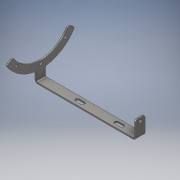
# Autodesk Inventor part: Bellmouth_union
Saved by Autodesk Inventor 2019 (Build 230136000, 136)
## iProperties
Created: 2021-06-28
Part Number: Bellmouth_union
Material: Stainless Steel
Document SubType Name: Sheet Metal
Designer: rtavi
Density: 8 g/cm^3
Sheet Metal Rule: Default_mm
Appearance: Semi-Polished
Mass: 21.766 g
Surface Area: 44.0313 cm^2
Volume: 2.72075 cm^3
Author: rtavi
Autodesk Inventor part; units mm, degrees
ref_plane "YZ Plane" through (0, 0, 0) normal (1, 0, 0) x (0, 1, 0)
ref_plane "XZ Plane" through (0, 0, 0) normal (0, 1, 0) x (-1, 0, 0)
ref_plane "XY Plane" through (0, 0, 0) normal (0, 0, 1) x (1, 0, 0)
sketch "Sketch1" plane through (0, 0, 0) normal (0, 1, 0) x (-1, 0, 0)
  arc A0 (33.3436, 28.8878) -> (33.3436, -28.8878) centre (52.2049, 0) ccw
  arc A1 (29.1632, 35.7118) -> (10.234, 6.6854) centre (52.2049, 0) ccw
  line L0 (33.9823, 31.5624) -> (31.9796, 35.0312)
  line L1 (33.9823, -31.5624) -> (31.9796, -35.0312)
  line L2 (134.5287, 0) -> (-168.388, 0) construction
  line L3 (8.2589, 5) -> (-106.7, 5)
  line L4 (-106.7, 5) -> (-106.7, -5) construction
  line L5 (-106.7, -5) -> (8.2589, -5)
  arc A2 (10, 5) -> (10, -5) centre (52.2049, 0) ccw construction
  arc A3 (10.234, -6.6854) -> (29.1632, -35.7118) centre (52.2049, 0) ccw
  circle A4 centre (14.7049, 0) radius 1.55
  circle A5 centre (25.6884, -26.5165) radius 1.55
  circle A6 centre (52.2049, -37.5) radius 1.55
  circle A7 centre (78.7214, -26.5165) radius 1.55
  circle A8 centre (89.7049, 0) radius 1.55
  circle A9 centre (78.7214, 26.5165) radius 1.55
  circle A10 centre (52.2049, 37.5) radius 1.55
  circle A11 centre (25.6884, 26.5165) radius 1.55
  line L6 (-82.1, -2.1) -> (-87.9, -2.1)
  line L7 (-90, 0) -> (-90, 0)
  line L8 (-87.9, 2.1) -> (-82.1, 2.1)
  line L9 (-80, 0) -> (-80, 0)
  arc A12 (-80, 0) -> (-82.1, 2.1) centre (-82.1, 0) ccw
  arc A13 (-82.1, -2.1) -> (-80, 0) centre (-82.1, 0) ccw
  arc A14 (-90, 0) -> (-87.9, -2.1) centre (-87.9, 0) ccw
  arc A15 (-87.9, 2.1) -> (-90, 0) centre (-87.9, 0) ccw
  arc A16 (-106.7, -3) -> (-104.7, -5) centre (-104.7, -3) ccw construction
  arc A17 (-104.7, 5) -> (-106.7, 3) centre (-104.7, 3) ccw construction
  arc A18 (29.1632, -35.7118) -> (31.9796, -35.0312) centre (30.2475, -34.0312) ccw
  arc A19 (33.9823, -31.5624) -> (33.3436, -28.8878) centre (32.2502, -30.5624) ccw
  arc A20 (33.3436, 28.8878) -> (33.9823, 31.5624) centre (32.2502, 30.5624) ccw
  arc A21 (31.9796, 35.0312) -> (29.1632, 35.7118) centre (30.2475, 34.0312) ccw
  arc A22 (8.2589, 5) -> (10.234, 6.6854) centre (8.2589, 7) ccw
  arc A23 (10.234, -6.6854) -> (8.2589, -5) centre (8.2589, -7) ccw
  line L10 (-47.6, 0) -> (-47.6, 0)
  arc A24 (-47.6, 0) -> (-45.5, -2.1) centre (-45.5, 0) ccw
  arc A25 (-45.5, 2.1) -> (-47.6, 0) centre (-45.5, 0) ccw
  line L11 (-37.6, 0) -> (-37.6, 0)
  arc A26 (-37.6, 0) -> (-39.7, 2.1) centre (-39.7, 0) ccw
  arc A27 (-39.7, -2.1) -> (-37.6, 0) centre (-39.7, 0) ccw
  line L12 (-45.5, 2.1) -> (-39.7, 2.1)
  line L13 (-39.7, -2.1) -> (-45.5, -2.1)
  line L14 (-124.7, -3) -> (-124.7, 3)
  line L15 (-106.7, -5) -> (-122.7, -5)
  line L16 (-122.7, 5) -> (-106.7, 5)
  arc A28 (-124.7, -3) -> (-122.7, -5) centre (-122.7, -3) ccw
  arc A29 (-122.7, 5) -> (-124.7, 3) centre (-122.7, 3) ccw
  line L17 (-121.1, -1.55) -> (-121.6, -1.55)
  line L18 (-123.15, 0) -> (-123.15, 0)
  line L19 (-121.6, 1.55) -> (-121.1, 1.55)
  line L20 (-119.55, 0) -> (-119.55, 0)
  arc A30 (-121.6, 1.55) -> (-123.15, 0) centre (-121.6, 0) ccw
  arc A31 (-123.15, 0) -> (-121.6, -1.55) centre (-121.6, 0) ccw
  arc A32 (-121.1, -1.55) -> (-119.55, 0) centre (-121.1, 0) ccw
  arc A33 (-119.55, 0) -> (-121.1, 1.55) centre (-121.1, 0) ccw
  point P0 (0, 0)
  point P1 (34.9549, 29.8779)
  point P2 (34.9549, -29.8779)
  point P3 (30.9549, 36.8061)
  point P4 (30.9549, -36.8061)
  point P5 (-80, -2.1)
  point P6 (-90, 2.1)
  point P7 (-90, -2.1)
  point P8 (-47.6, 2.1)
  point P9 (-47.6, -2.1)
  point P10 (-37.6, -2.1)
  point P11 (-123.15, 1.55)
  point P12 (-123.15, -1.55)
  dimension "d0" = 34.5
  dimension "d1" = 42.5
  dimension "d2" = 8
  dimension "d3" = 8
  dimension "d4" = 120
  dimension "d5" = 10
  dimension "d6" = 10
  dimension "d15" = 3.1
  dimension "d16" = 37.5
  dimension "d19" = 360
  dimension "d21" = 4.2
  dimension "d22" = 10
  dimension "d23" = 16.7
  dimension "d24" = 2.1
  dimension "d25" = 2
  dimension "d28" = 42.4
  dimension "d33" = 18
  dimension "d34" = 2
  dimension "d43" = 3.1
  dimension "d44" = 1.55
  dimension "d45" = 1.55
  dimension "d46" = 0.5
  dimension "d47" = 90
  measures "d0" radius of A0
  measures "d1" radius of A1
  measures "d2" distance of point (34.955, 29.878) point (30.955, 36.806)
  measures "d3" distance of point (34.955, -29.878) point (30.955, -36.806)
  measures "d4" angle of L1 L0
  measures "d5" distance of L3.end L4.end
  measures "d6" horizontal distance of A2.start point (0, 0)
  measures "d15" diameter of A4
  measures "d16" distance of A0.centre A4.centre
  measures "d21" distance of point (-90, -2.1) point (-90, 2.1)
  measures "d22" distance of point (-80, -2.1) point (-90, -2.1)
  measures "d23" distance between parallel lines of L4 L7
  measures "d24" radius of A12
  measures "d25" radius of A16
  measures "d28" distance of point (-90, 2.1) point (-47.6, 2.1)
  measures "d33" distance between parallel lines of L4 L14
  measures "d34" radius of A28
  measures "d43" distance of point (-123.15, -1.55) point (-123.15, 1.55)
  measures "d44" distance between parallel lines of L18 L14
  measures "d45" radius of A30
  measures "d46" distance of A32.centre A31.centre
  measures "d47" horizontal distance of point (-90, 2.1) point (0, 0)
extrude "Plate1" add sketch "Sketch1" against normal blind 1.5 contours A0 A19 L1 A18 A3 A23 L5 L15 A28 L14 A29 L16 L3 A22 A1 A21 L0 A20
sketch "Sketch2" plane through (0, 0, 0) normal (0, 1, 0) x (-1, 0, 0)
  line L0 (0, -7) -> (0, 7) construction
  line L1 (-122.7, 5) -> (8.2589, 5) construction
  line L2 (0, 5) -> (0, -5)
  point P0 (0, 0)
  point P1 (-70, 5)
  point P2 (30, 5)
  point P3 (-93, 5)
  constraints: 3 point on line, 2 end point
fold "Fold1" angle 90 bend radius 1.5 thickness 1.5 k factor 0.44 line from (0, 0, 5) to (0, 0, -5) line at bend centre moving side (-1, 0, 0) folds toward (0, 1, 0)
sketch "Sketch3" plane through (0, 0, 0) normal (0, 1, 0) x (-1, 0, 0)
  line L0 (-106.7, 5) -> (-106.7, -5) construction
  point P0 (0, 0)
fold "Fold2" angle 90 bend radius 1.5 thickness 1.5 k factor 0.44 line from (106.7, 0, 5) to (106.7, 0, -5) line at bend centre moving side (1, 0, 0) folds toward (0, 1, 0)
equation "\"d8\" = Thickness"
equation "\"d9\" = BendReliefWidth"
equation "\"d10\" = BendReliefDepth"
equation "\"d11\" = MinimumRemnant"
equation "\"d12\" = TransitionRadius"
equation "\"d14\" = BendRadius"
equation "\"d37\" = BendReliefWidth"
equation "\"d38\" = BendReliefDepth"
equation "\"d39\" = MinimumRemnant"
equation "\"d40\" = TransitionRadius"
equation "\"d42\" = BendRadius"
equation "\"BendRadius\" = Thickness"
equation "\"BendReliefWidth\" = Thickness"
equation "\"BendReliefDepth\" = 0.5 * Thickness"
equation "\"CornerReliefSize\" = 4 * Thickness"
equation "\"MinimumRemnant\" = 2 * Thickness"
equation "\"TransitionRadius\" = BendRadius"
equation "\"JacobiRadiusSize\" = BendRadius"
equation "\"GapSize\" = Thickness"
equation "\"Thickness\" = 1.5"
body "Solid1"
